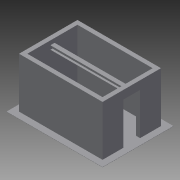
# Autodesk Inventor part: SP_AST_Compartment_Drawing
Saved by Autodesk Inventor 2013 SP2 (Build 170200200, 200)
## iProperties
Created: 2014-01-15
Part Number: SP_AST_Compartment_Drawing
Material: Generic
Document SubType Name: Modeling
Designer: mcgratta
Density: 1 g/cm^3
Author: mcgratta
Autodesk Inventor part; units mm, degrees
ref_plane "YZ Plane" through (0, 0, 0) normal (1, 0, 0) x (0, 1, 0)
ref_plane "XZ Plane" through (0, 0, 0) normal (0, 1, 0) x (-1, 0, 0)
ref_plane "XY Plane" through (0, 0, 0) normal (0, 0, 1) x (1, 0, 0)
sketch "Sketch1" plane through (0, 0, 0) normal (0, 1, 0) x (-1, 0, 0)
  line L0 (500, 500) -> (-4100, 500)
  line L1 (-4100, 500) -> (-4100, -2900)
  line L2 (-4100, -2900) -> (500, -2900)
  line L3 (500, -2900) -> (500, 500)
  point P0 (0, 0)
  dimension "d0" = 4600
  dimension "d1" = 500
  dimension "d2" = 500
  dimension "d3" = 3400
  constraints: 8 end point, 2 parallel, 1 horizontal, 1 perpendicular
  measures "d0" distance between parallel lines of L1 L3
  measures "d1" distance from line of point (0, 0) L3
  measures "d2" distance from line of L0 point (0, 0)
  measures "d3" distance between parallel lines of L0 L2
extrude "Extrusion1" add sketch "Sketch1" along normal blind 10
sketch "Sketch2" plane through (0, 10, 0) normal (0, 1, 0) x (1, 0, 0)
  line L0 (-500, -500) -> (4100, -500) projected
  line L1 (-500, 2900) -> (-500, -500) projected
  line L2 (-200, -200) -> (0, -200)
  line L3 (0, -200) -> (0, 2600)
  line L4 (0, 2600) -> (-200, 2600)
  line L5 (-200, 2600) -> (-200, -200)
  point P0 (0, 0)
  dimension "d6" = 300
  dimension "d7" = 2800
  dimension "d8" = 200
  dimension "d9" = 300
  constraints: 8 end point, 2 parallel, 1 horizontal, 1 perpendicular
  measures "d6" distance between parallel lines of L0 L2
  measures "d7" distance between parallel lines of L4 L2
  measures "d8" distance between parallel lines of L3 L5
  measures "d9" distance between parallel lines of L5 L1
extrude "Extrusion2" add sketch "Sketch2" along normal blind 2400
sketch "Sketch3" plane through (0, 10, 0) normal (0, 1, 0) x (1, 0, 0)
  line L0 (0, 2600) -> (0, -200) projected
  line L1 (-500, -500) -> (4100, -500) projected
  line L2 (0, -200) -> (3600, -200)
  line L3 (3600, -200) -> (3600, 0)
  line L4 (3600, 0) -> (0, 0)
  line L5 (0, 0) -> (0, -200)
  point P0 (0, 0)
  dimension "d12" = 300
  dimension "d13" = 200
  dimension "d14" = 3600
  constraints: 8 end point, 2 parallel, 1 horizontal, 1 perpendicular
  measures "d12" distance between parallel lines of L1 L2
  measures "d13" distance between parallel lines of L2 L4
  measures "d14" distance between parallel lines of L3 L0
extrude "Extrusion3" add sketch "Sketch3" along normal blind 2400
sketch "Sketch4" plane through (0, 10, 0) normal (0, 1, 0) x (1, 0, 0)
  line L0 (4100, 2900) -> (-500, 2900) projected
  line L1 (0, 2600) -> (0, 0) projected
  line L2 (0, 2600) -> (3600, 2600)
  line L3 (3600, 2600) -> (3600, 2400)
  line L4 (3600, 2400) -> (0, 2400)
  line L5 (0, 2400) -> (0, 2600)
  dimension "d17" = 300
  dimension "d18" = 200
  dimension "d19" = 3600
  constraints: 8 end point, 2 parallel, 1 horizontal, 1 perpendicular
  measures "d17" distance between parallel lines of L2 L0
  measures "d18" distance between parallel lines of L4 L2
  measures "d19" distance between parallel lines of L3 L1
extrude "Extrusion4" add sketch "Sketch4" along normal blind 2400
sketch "Sketch5" plane through (0, 10, 0) normal (0, 1, 0) x (1, 0, 0)
  line L0 (3600, -200) -> (3800, -200)
  line L1 (3800, -200) -> (3800, 2600)
  line L2 (3800, 2600) -> (3600, 2600)
  line L3 (3600, 2600) -> (3600, -200)
  dimension "d22" = 200
  dimension "d24" = 2800
  constraints: 8 end point, 2 parallel, 1 horizontal, 1 perpendicular
  measures "d22" distance between parallel lines of L1 L3
  measures "d24" distance between parallel lines of L0 L2
extrude "Extrusion5" add sketch "Sketch5" along normal blind 2400
sketch "Sketch6" plane through (3800, 10, 200) normal (1, 0, 0) x (0, 0, -1)
  line L0 (2800, 0) -> (0, 0) projected
  line L1 (2800, 0) -> (2800, 2400) projected
  line L2 (1000, 0) -> (1800, 0)
  line L3 (1800, 0) -> (1800, 2000)
  line L4 (1800, 2000) -> (1000, 2000)
  line L5 (1000, 2000) -> (1000, 0)
  point P0 (200, -10)
  dimension "d27" = 800
  dimension "d29" = 2000
  dimension "d30" = 1000
  constraints: 8 end point, 2 parallel, 1 horizontal, 1 perpendicular, 1 point on line
  measures "d27" distance between parallel lines of L3 L5
  measures "d29" distance between parallel lines of L0 L4
  measures "d30" distance between parallel lines of L1 L3
extrude "Extrusion6" cut sketch "Sketch6" along normal blind 100 and the other way blind 300
sketch "Sketch8" plane through (0, 10, 0) normal (1, 0, 0) x (0, 0, -1)
  line L0 (0, 2400) -> (0, 0) projected
  line L1 (2400, 0) -> (0, 0) projected
  line L2 (1200, 2185) -> (1209, 2185)
  line L3 (1209, 2185) -> (1209, 2015)
  line L4 (1209, 2015) -> (1200, 2015)
  line L5 (1200, 2015) -> (1200, 2185)
  line L6 (1104.5, 2200) -> (1304.5, 2200)
  line L7 (1304.5, 2200) -> (1304.5, 2185)
  line L8 (1304.5, 2185) -> (1104.5, 2185)
  line L9 (1104.5, 2185) -> (1104.5, 2200)
  line L10 (1104.5, 2015) -> (1304.5, 2015)
  line L11 (1304.5, 2015) -> (1304.5, 2000)
  line L12 (1304.5, 2000) -> (1104.5, 2000)
  line L13 (1104.5, 2000) -> (1104.5, 2015)
  point P0 (0, -10)
  dimension "d35" = 9
  dimension "d37" = 1200
  dimension "d38" = 170
  dimension "d39" = 2015
  dimension "d40" = 95.5
  dimension "d41" = 95.5
  dimension "d42" = 15
  dimension "d43" = 15
  dimension "d44" = 0
  dimension "d45" = 200
  constraints: 24 end point, 6 parallel, 3 horizontal, 3 perpendicular
  measures "d35" distance between parallel lines of L3 L5
  measures "d37" distance between parallel lines of L5 L0
  measures "d38" distance between parallel lines of L4 L2
  measures "d39" distance from line of L1 L4.end
  measures "d40" distance between parallel lines of L7 L3
  measures "d41" distance between parallel lines of L9 L5
  measures "d42" distance between parallel lines of L8 L6
  measures "d43" distance between parallel lines of L12 L10
  measures "d44" distance between parallel lines of L10 L4
  measures "d45" distance of L11.end L12.end
extrude "Extrusion7" add sketch "Sketch8" along normal blind 3600
sketch "Sketch9" plane through (0, 10, 0) normal (0, 1, 0) x (1, 0, 0)
  line L0 (0, 2400) -> (0, 0) projected
  line L1 (0, 0) -> (3600, 0) projected
  line L2 (25, 325) -> (325, 325)
  line L3 (325, 325) -> (325, 25)
  line L4 (325, 25) -> (25, 25)
  line L5 (25, 25) -> (25, 325)
  dimension "d48" = 25
  dimension "d49" = 25
  dimension "d50" = 300
  dimension "d51" = 300
  constraints: 8 end point, 2 parallel, 1 horizontal, 1 perpendicular
  measures "d48" distance between parallel lines of L0 L5
  measures "d49" distance between parallel lines of L1 L4
  measures "d50" distance between parallel lines of L4 L2
  measures "d51" distance between parallel lines of L3 L5
extrude "Extrusion8" add sketch "Sketch9" along normal blind 650
body "Solid1"
